Autodesk Inventor part; units mm, degrees
(part 2 of 2)
  spline S24 degree 3 poles (37.9264, 36.6557) (37.8142, 36.6489) (37.5899, 36.6355) (37.2542, 36.6053) (36.9192, 36.5675) (36.5853, 36.521) (36.2528, 36.4655) (35.922, 36.4003) (35.5935, 36.3248) (35.2677, 36.238) (34.9991, 36.1554) (34.7866, 36.0823) (34.6286, 36.0236) (34.4721, 35.9609) (34.3182, 35.8924) (34.1905, 35.8338) (34.0853, 35.7941) (34.005, 35.7686) (33.9236, 35.7466) (33.8411, 35.7292) (33.7576, 35.7173) (33.6735, 35.7113) (33.5891, 35.7119) (33.5051, 35.7192) (33.422, 35.734) (33.3408, 35.757) (33.2622, 35.7876) (33.1864, 35.8246) (33.1155, 35.8705) (33.0495, 35.923) (32.9887, 35.9816) (32.9188, 36.0698) (32.8387, 36.1852) (32.7537, 36.297) (32.6914, 36.3907) (32.6544, 36.4666) (32.6249, 36.5456) (32.6031, 36.6272) (32.5912, 36.7107) (32.5864, 36.7949) (32.5896, 36.8793) (32.6012, 36.9629) (32.6201, 37.0451) (32.6457, 37.1255) (32.6773, 37.2036) (32.7144, 37.2794) (32.7564, 37.3525) (32.8025, 37.4231) (32.8514, 37.4917) (32.9217, 37.5794) (33.0168, 37.6828) (33.1295, 37.8081) (33.2374, 37.9376) (33.3421, 38.0698) (33.4772, 38.2493) (33.6387, 38.4793) (33.8217, 38.7624) (33.995, 39.0516) (34.1591, 39.3461) (34.3145, 39.6452) (34.4618, 39.9484) (34.6012, 40.2554) (34.7335, 40.5654) (34.8155, 40.7747) (34.8565, 40.8793) knots -1.078574 -1.078574 -1.078574 -1.078574 -1.044867 -1.011159 -0.977452 -0.943745 -0.910038 -0.876331 -0.842624 -0.808918 -0.775212 -0.758359 -0.741505 -0.724651 -0.707798 -0.690947 -0.68252 -0.674093 -0.665668 -0.657242 -0.648815 -0.640389 -0.631963 -0.623537 -0.61511 -0.606685 -0.598264 -0.589839 -0.581413 -0.57299 -0.564565 -0.556141 -0.539287 -0.522433 -0.514009 -0.505584 -0.49716 -0.488735 -0.48031 -0.471889 -0.463464 -0.455037 -0.446611 -0.438185 -0.429758 -0.421332 -0.412906 -0.40448 -0.396053 -0.387627 -0.370775 -0.353922 -0.337069 -0.320215 -0.303361 -0.269656 -0.235949 -0.202243 -0.168536 -0.134829 -0.101122 -0.067415 -0.033707 0 0 0 0 construction
  arc A24 (34.8565, 40.8793) -> (33.8695, 41.975) centre (10.5928, 20.0161) ccw construction
  spline S25 degree 3 poles (33.8695, 41.975) (33.7612, 41.9451) (33.5446, 41.8854) (33.2224, 41.786) (32.9026, 41.6794) (32.5857, 41.5645) (32.272, 41.441) (31.9621, 41.3085) (31.6564, 41.1663) (31.3558, 41.0137) (31.1103, 40.8771) (30.9176, 40.7614) (30.7753, 40.6711) (30.6352, 40.5773) (30.4989, 40.4782) (30.3861, 40.3944) (30.2915, 40.3336) (30.2182, 40.2921) (30.1432, 40.2536) (30.0661, 40.2195) (29.9869, 40.1904) (29.9059, 40.1671) (29.8233, 40.1501) (29.7395, 40.1398) (29.6552, 40.137) (29.571, 40.1426) (29.4878, 40.1562) (29.4059, 40.1766) (29.327, 40.2068) (29.2515, 40.2444) (29.1799, 40.2891) (29.0932, 40.3608) (28.9908, 40.457) (28.8844, 40.5487) (28.804, 40.6274) (28.752, 40.694) (28.7067, 40.7651) (28.6684, 40.8404) (28.6395, 40.9197) (28.6173, 41.001) (28.6029, 41.0842) (28.5968, 41.1683) (28.5982, 41.2527) (28.6065, 41.3366) (28.6212, 41.4197) (28.6418, 41.5015) (28.6676, 41.5817) (28.698, 41.6603) (28.7317, 41.7376) (28.7822, 41.838) (28.8537, 41.959) (28.9379, 42.105) (29.0165, 42.2541) (29.0914, 42.4051) (29.1862, 42.6088) (29.2964, 42.8673) (29.4166, 43.1823) (29.5259, 43.5012) (29.6252, 43.8234) (29.7151, 44.1483) (29.7961, 44.4755) (29.8685, 44.8047) (29.9336, 45.1355) (29.9703, 45.3572) (29.9886, 45.4681) knots -1.078574 -1.078574 -1.078574 -1.078574 -1.044867 -1.011159 -0.977452 -0.943745 -0.910038 -0.876331 -0.842624 -0.808918 -0.775212 -0.758359 -0.741505 -0.724651 -0.707798 -0.690947 -0.68252 -0.674093 -0.665668 -0.657242 -0.648815 -0.640389 -0.631963 -0.623537 -0.61511 -0.606685 -0.598264 -0.589839 -0.581413 -0.57299 -0.564565 -0.556141 -0.539287 -0.522433 -0.514009 -0.505584 -0.49716 -0.488735 -0.48031 -0.471889 -0.463464 -0.455037 -0.446611 -0.438185 -0.429758 -0.421332 -0.412906 -0.40448 -0.396053 -0.387627 -0.370775 -0.353922 -0.337069 -0.320215 -0.303361 -0.269656 -0.235949 -0.202243 -0.168536 -0.134829 -0.101122 -0.067415 -0.033707 0 0 0 0 construction
  arc A25 (29.9886, 45.4681) -> (28.7954, 46.3347) centre (10.5928, 20.0161) ccw construction
  spline S26 degree 3 poles (28.7954, 46.3347) (28.6956, 46.2829) (28.4962, 46.1794) (28.2017, 46.0153) (27.9111, 45.8445) (27.625, 45.6662) (27.3438, 45.4802) (27.0682, 45.2861) (26.7987, 45.0835) (26.5364, 44.8717) (26.3247, 44.687) (26.1603, 44.5338) (26.0398, 44.4159) (25.9223, 44.295) (25.8096, 44.1698) (25.7167, 44.0644) (25.6368, 43.9853) (25.5737, 43.9293) (25.5084, 43.8761) (25.4401, 43.8267) (25.3686, 43.7819) (25.2942, 43.7422) (25.217, 43.7083) (25.1372, 43.6809) (25.0553, 43.6606) (24.9717, 43.6486) (24.8875, 43.6445) (24.8032, 43.6475) (24.7198, 43.6607) (24.6381, 43.6817) (24.5587, 43.7106) (24.459, 43.7627) (24.3389, 43.8355) (24.2158, 43.9031) (24.1207, 43.9633) (24.056, 44.0176) (23.9969, 44.0778) (23.9438, 44.1435) (23.899, 44.215) (23.8604, 44.2899) (23.829, 44.3683) (23.8056, 44.4493) (23.7894, 44.5321) (23.7801, 44.616) (23.7772, 44.7003) (23.7803, 44.7845) (23.7889, 44.8684) (23.8023, 44.9516) (23.8191, 45.0342) (23.8477, 45.143) (23.8925, 45.2761) (23.9445, 45.4364) (23.9904, 45.5986) (24.0322, 45.7619) (24.0826, 45.9809) (24.1366, 46.2566) (24.1887, 46.5897) (24.2293, 46.9244) (24.2595, 47.2602) (24.2798, 47.5967) (24.2911, 47.9336) (24.2935, 48.2707) (24.2883, 48.6078) (24.2781, 48.8323) (24.273, 48.9445) knots -1.078574 -1.078574 -1.078574 -1.078574 -1.044867 -1.011159 -0.977452 -0.943745 -0.910038 -0.876331 -0.842624 -0.808918 -0.775212 -0.758359 -0.741505 -0.724651 -0.707798 -0.690947 -0.68252 -0.674093 -0.665668 -0.657242 -0.648815 -0.640389 -0.631963 -0.623537 -0.61511 -0.606685 -0.598264 -0.589839 -0.581413 -0.57299 -0.564565 -0.556141 -0.539287 -0.522433 -0.514009 -0.505584 -0.49716 -0.488735 -0.48031 -0.471889 -0.463464 -0.455037 -0.446611 -0.438185 -0.429758 -0.421332 -0.412906 -0.40448 -0.396053 -0.387627 -0.370775 -0.353922 -0.337069 -0.320215 -0.303361 -0.269656 -0.235949 -0.202243 -0.168536 -0.134829 -0.101122 -0.067415 -0.033707 0 0 0 0 construction
  arc A26 (24.273, 48.9445) -> (22.9257, 49.5441) centre (10.5928, 20.0161) ccw construction
  spline S27 degree 3 poles (22.9257, 49.5441) (22.8389, 49.4727) (22.6653, 49.33) (22.4114, 49.1082) (22.1626, 48.8808) (21.9198, 48.6469) (21.6835, 48.4065) (21.4542, 48.1593) (21.2328, 47.9051) (21.0202, 47.6434) (20.8515, 47.4188) (20.7225, 47.2347) (20.6293, 47.0943) (20.5395, 46.9516) (20.4552, 46.8057) (20.3863, 46.6833) (20.3246, 46.5893) (20.2745, 46.5215) (20.2217, 46.4558) (20.1651, 46.3933) (20.1046, 46.3346) (20.04, 46.2803) (19.9715, 46.2311) (19.8992, 46.1877) (19.8232, 46.1509) (19.7441, 46.1217) (19.6625, 46.1002) (19.5794, 46.0856) (19.4951, 46.0811) (19.4108, 46.0848) (19.3272, 46.0965) (19.2188, 46.1267) (19.0861, 46.1729) (18.9517, 46.2134) (18.8462, 46.2526) (18.7716, 46.2923) (18.7013, 46.3389) (18.6357, 46.392) (18.577, 46.4527) (18.5237, 46.518) (18.4767, 46.5881) (18.4369, 46.6625) (18.4039, 46.7401) (18.3773, 46.8202) (18.357, 46.902) (18.3425, 46.9851) (18.3334, 47.069) (18.3292, 47.1531) (18.3285, 47.2374) (18.3339, 47.3497) (18.35, 47.4893) (18.3675, 47.6569) (18.3787, 47.8251) (18.3857, 47.9935) (18.3894, 48.2182) (18.3849, 48.4991) (18.3666, 48.8358) (18.3368, 49.1716) (18.2965, 49.5063) (18.2464, 49.8396) (18.1873, 50.1715) (18.1196, 50.5018) (18.0445, 50.8304) (17.9878, 51.0479) (17.9595, 51.1566) knots -1.078574 -1.078574 -1.078574 -1.078574 -1.044867 -1.011159 -0.977452 -0.943745 -0.910038 -0.876331 -0.842624 -0.808918 -0.775212 -0.758359 -0.741505 -0.724651 -0.707798 -0.690947 -0.68252 -0.674093 -0.665668 -0.657242 -0.648815 -0.640389 -0.631963 -0.623537 -0.61511 -0.606685 -0.598264 -0.589839 -0.581413 -0.57299 -0.564565 -0.556141 -0.539287 -0.522433 -0.514009 -0.505584 -0.49716 -0.488735 -0.48031 -0.471889 -0.463464 -0.455037 -0.446611 -0.438185 -0.429758 -0.421332 -0.412906 -0.40448 -0.396053 -0.387627 -0.370775 -0.353922 -0.337069 -0.320215 -0.303361 -0.269656 -0.235949 -0.202243 -0.168536 -0.134829 -0.101122 -0.067415 -0.033707 0 0 0 0 construction
  arc A27 (17.9595, 51.1566) -> (16.517, 51.463) centre (10.5928, 20.0161) ccw construction
  spline S28 degree 3 poles (16.517, 51.463) (16.4469, 51.3751) (16.3068, 51.1994) (16.1045, 50.9297) (15.9085, 50.6555) (15.7196, 50.3762) (15.5384, 50.092) (15.3655, 49.8025) (15.2018, 49.5078) (15.0483, 49.2077) (14.93, 48.9528) (14.8421, 48.746) (14.7801, 48.5893) (14.7219, 48.4311) (14.6698, 48.2708) (14.6279, 48.1367) (14.5871, 48.032) (14.5522, 47.9552) (14.5141, 47.88) (14.4718, 47.8071) (14.4248, 47.7371) (14.373, 47.6705) (14.3161, 47.6082) (14.2544, 47.5507) (14.1878, 47.4989) (14.1164, 47.4539) (14.0411, 47.4159) (13.9628, 47.3844) (13.8813, 47.3624) (13.7981, 47.3485) (13.7139, 47.3425) (13.6016, 47.3496) (13.4622, 47.3672) (13.3223, 47.3789) (13.211, 47.3953) (13.1298, 47.4186) (13.0513, 47.4495) (12.9761, 47.4879) (12.9061, 47.535) (12.8403, 47.5878) (12.7798, 47.6466) (12.7254, 47.7111) (12.677, 47.7802) (12.6343, 47.8529) (12.5974, 47.9288) (12.5659, 48.007) (12.5397, 48.0871) (12.5181, 48.1686) (12.4999, 48.2509) (12.4817, 48.3619) (12.4685, 48.5017) (12.4508, 48.6693) (12.4267, 48.8362) (12.3986, 49.0024) (12.3555, 49.2229) (12.2927, 49.4968) (12.2048, 49.8223) (12.1058, 50.1445) (11.9968, 50.4635) (11.8785, 50.7792) (11.7517, 51.0916) (11.6168, 51.4005) (11.475, 51.7063) (11.3744, 51.9073) (11.3241, 52.0077) knots -1.078574 -1.078574 -1.078574 -1.078574 -1.044867 -1.011159 -0.977452 -0.943745 -0.910038 -0.876331 -0.842624 -0.808918 -0.775212 -0.758359 -0.741505 -0.724651 -0.707798 -0.690947 -0.68252 -0.674093 -0.665668 -0.657242 -0.648815 -0.640389 -0.631963 -0.623537 -0.61511 -0.606685 -0.598264 -0.589839 -0.581413 -0.57299 -0.564565 -0.556141 -0.539287 -0.522433 -0.514009 -0.505584 -0.49716 -0.488735 -0.48031 -0.471889 -0.463464 -0.455037 -0.446611 -0.438185 -0.429758 -0.421332 -0.412906 -0.40448 -0.396053 -0.387627 -0.370775 -0.353922 -0.337069 -0.320215 -0.303361 -0.269656 -0.235949 -0.202243 -0.168536 -0.134829 -0.101122 -0.067415 -0.033707 0 0 0 0 construction
  arc A28 (11.3241, 52.0077) -> (9.8493, 52.0075) centre (10.5928, 20.0161) ccw construction
  spline S29 degree 3 poles (9.8493, 52.0075) (9.7991, 51.907) (9.6985, 51.706) (9.5568, 51.4001) (9.422, 51.0911) (9.2954, 50.7787) (9.1772, 50.463) (9.0683, 50.1439) (8.9694, 49.8216) (8.8817, 49.4961) (8.8189, 49.2223) (8.776, 49.0017) (8.7479, 48.8355) (8.7239, 48.6686) (8.7062, 48.501) (8.6931, 48.3611) (8.675, 48.2502) (8.6568, 48.1679) (8.6352, 48.0864) (8.609, 48.0063) (8.5776, 47.928) (8.5407, 47.8522) (8.4981, 47.7794) (8.4496, 47.7103) (8.3953, 47.6457) (8.3348, 47.5869) (8.269, 47.5341) (8.199, 47.487) (8.1238, 47.4486) (8.0454, 47.4176) (7.9642, 47.3943) (7.8529, 47.3778) (7.7129, 47.3661) (7.5736, 47.3484) (7.4613, 47.3413) (7.377, 47.3473) (7.2939, 47.3612) (7.2123, 47.3831) (7.134, 47.4146) (7.0587, 47.4525) (6.9873, 47.4975) (6.9207, 47.5493) (6.8589, 47.6068) (6.8021, 47.6691) (6.7502, 47.7356) (6.7032, 47.8056) (6.6608, 47.8785) (6.6228, 47.9537) (6.5878, 48.0304) (6.547, 48.1352) (6.505, 48.2692) (6.4529, 48.4295) (6.3946, 48.5877) (6.3325, 48.7444) (6.2446, 48.9512) (6.1262, 49.206) (5.9725, 49.5061) (5.8087, 49.8007) (5.6357, 50.0901) (5.4544, 50.3743) (5.2654, 50.6535) (5.0693, 50.9276) (4.8669, 51.1972) (4.7267, 51.3729) (4.6566, 51.4607) knots -1.078574 -1.078574 -1.078574 -1.078574 -1.044867 -1.011159 -0.977452 -0.943745 -0.910038 -0.876331 -0.842624 -0.808918 -0.775212 -0.758359 -0.741505 -0.724651 -0.707798 -0.690947 -0.68252 -0.674093 -0.665668 -0.657242 -0.648815 -0.640389 -0.631963 -0.623537 -0.61511 -0.606685 -0.598264 -0.589839 -0.581413 -0.57299 -0.564565 -0.556141 -0.539287 -0.522433 -0.514009 -0.505584 -0.49716 -0.488735 -0.48031 -0.471889 -0.463464 -0.455037 -0.446611 -0.438185 -0.429758 -0.421332 -0.412906 -0.40448 -0.396053 -0.387627 -0.370775 -0.353922 -0.337069 -0.320215 -0.303361 -0.269656 -0.235949 -0.202243 -0.168536 -0.134829 -0.101122 -0.067415 -0.033707 0 0 0 0 construction
  arc A29 (4.6566, 51.4607) -> (3.2142, 51.1538) centre (10.5928, 20.0161) ccw construction
  circle A30 centre (10.5928, 20.0161) radius 6.16 construction
  line L0 (27.8335, 2.609) -> (17.5359, 14.0412) construction
  arc A31 (17.5359, 14.0412) -> (19.3648, 22.6538) centre (10.5928, 20.0161) ccw construction
  line L1 (19.3648, 22.6538) -> (33.4197, 28.9146) construction
  arc A32 (27.8335, 2.609) -> (33.4197, 28.9146) centre (10.5928, 20.0161) ccw construction
  line L2 (-0.6347, -1.7599) -> (7.0559, 11.5665) construction
  arc A33 (7.0559, 11.5665) -> (15.8121, 12.4885) centre (10.5928, 20.0161) ccw construction
  line L3 (15.8121, 12.4885) -> (26.1097, 1.0562) construction
  arc A34 (-0.6347, -1.7599) -> (26.1097, 1.0562) centre (10.5928, 20.0161) ccw construction
  line L4 (6.8765, 44.2326) -> (8.4877, 28.9309) construction
  arc A35 (8.4877, 28.9309) -> (1.9457, 23.0382) centre (10.5928, 20.0161) ccw construction
  line L5 (1.9457, 23.0382) -> (-13.1049, 26.2343) construction
  arc A36 (6.8765, 44.2326) -> (-13.1049, 26.2343) centre (10.5928, 20.0161) ccw construction
  line L6 (10.7949, 29.1739) -> (9.1837, 44.4755) construction
  arc A37 (32.4757, 31.0339) -> (9.1837, 44.4755) centre (10.5928, 20.0161) ccw construction
  line L7 (32.4757, 31.0339) -> (18.4208, 24.773) construction
  arc A38 (18.4208, 24.773) -> (10.7949, 29.1739) centre (10.5928, 20.0161) ccw construction
  line L8 (-13.5869, 23.965) -> (1.4638, 20.7688) construction
  arc A39 (1.4638, 20.7688) -> (5.0465, 12.7261) centre (10.5928, 20.0161) ccw construction
  line L9 (5.0465, 12.7261) -> (-2.6441, -0.6003) construction
  arc A40 (-13.5869, 23.965) -> (-2.6441, -0.6003) centre (10.5928, 20.0161) ccw construction
  circle A41 centre (10.5928, 20.0161) radius 5.86 construction
  circle A42 centre (10.5928, 20.0161) radius 3.86 construction
  circle A43 centre (10.5928, 20.0161) radius 6.36
  circle A44 centre (10.5928, 20.0161) radius 9.16
  point P0 (7.7432, 45.9796)
  dimension "d0" = 0.5
  constraints: 2 centre point, 1 coincident, 1 concentric
  measures "d0" radial gap between concentric circles of A41 A43
extrude "Extrusion1" add sketch "Sketch1" along normal blind 5.5
body "Solid1"
